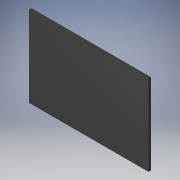
# Autodesk Inventor part: BA12
Saved by Autodesk Inventor 2017 (Build 210142000, 142)
## iProperties
Created: 2018-10-18
Part Number: BA12
Material: ABS Plastic
Document SubType Name: Modeling
Designer: Dell
Density: 1.06 g/cm^3
Appearance: Smooth - Black
Author: Dell
Autodesk Inventor part; units mm, degrees
ref_plane "YZ Plane" through (0, 0, 0) normal (1, 0, 0) x (0, 1, 0)
ref_plane "XZ Plane" through (0, 0, 0) normal (0, 1, 0) x (-1, 0, 0)
ref_plane "XY Plane" through (0, 0, 0) normal (0, 0, 1) x (1, 0, 0)
sketch "Sketch1" plane through (0, 0, 0) normal (0, 0, 1) x (1, 0, 0)
  line L0 (0, 0) -> (525.78, 0)
  line L1 (525.78, 0) -> (525.78, 355.6)
  line L2 (525.78, 355.6) -> (0, 355.6)
  line L3 (0, 355.6) -> (0, 0)
  dimension "d0" = 525.78
  dimension "d1" = 355.6
  constraints: 8 end point, 2 parallel, 1 horizontal, 1 perpendicular
  measures "d0" distance of L2.end L1.end
  measures "d1" distance of L1.end L0.end
extrude "Extrusion1" add sketch "Sketch1" along normal blind 10
sketch "Sketch6" plane through (0, 0, 10) normal (0, 0, 1) x (1, 0, 0)
  circle A0 centre (327.348, 311.15) radius 2.3812
  circle A1 centre (390.848, 311.15) radius 2.3813
  line L0 (327.348, 311.15) -> (390.848, 311.15) construction
  line L1 (314.648, 355.6) -> (403.548, 355.6) construction
  line L2 (403.548, 355.6) -> (403.548, 266.7) construction
  line L3 (403.548, 266.7) -> (314.648, 266.7) construction
  line L4 (314.648, 266.7) -> (314.648, 355.6) construction
  line L5 (525.78, 0) -> (525.78, 355.6) projected
  line L6 (525.78, 355.6) -> (0, 355.6) projected
  point P0 (0, 0)
  point P1 (359.098, 311.15)
  point P2 (359.098, 355.6)
  point P3 (314.648, 311.15)
  point P4 (359.098, 266.7)
  dimension "d20" = 4.7625
  dimension "d21" = 4.7625
  dimension "d22" = 63.5
  dimension "d23" = 88.9
  dimension "d25" = 88.9
  dimension "d26" = 122.232
  constraints: 10 end point, 4 midpoint, 2 centre point, 2 horizontal, 2 parallel, 1 horizontal alignment, 1 perpendicular, 1 point on line, 1 vertical alignment
  measures "d20" diameter of A0
  measures "d21" diameter of A1
  measures "d22" distance of L0.start L0.end
  measures "d23" distance of L1.start L1.end
  measures "d25" distance of L3.end L1.start
  measures "d26" distance between parallel lines of L5 L2
extrude "Extrusion4" cut sketch "Sketch6" against normal through all
body "Solid1"
